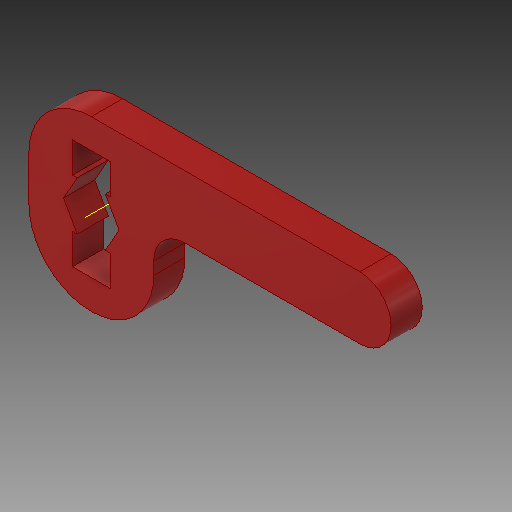
# Autodesk Inventor part: В. шарн. - держатель соединителя
Saved by Autodesk Inventor 2018 (Build 220112000, 112)
## iProperties
Created: 2020-02-23
Part Number: В. шарн. - держатель соединителя
Material: Типовые
Document SubType Name: Modeling
Designer: Leancher
Density: 1 g/cm^3
Appearance: По умолчанию
Author: Leancher
Autodesk Inventor part; units mm, degrees
ref_plane "YZ Plane" through (0, 0, 0) normal (1, 0, 0) x (0, 1, 0)
ref_plane "XZ Plane" through (0, 0, 0) normal (0, 1, 0) x (-1, 0, 0)
ref_plane "XY Plane" through (0, 0, 0) normal (0, 0, 1) x (1, 0, 0)
sketch "Эскиз1" plane through (0, 0, 0) normal (0, 0, 1) x (1, 0, 0)
  arc A0 (5.088, 16.8311) -> (-4.912, 6.8311) centre (5.088, 6.8311) ccw
  line L0 (7.3397, 7.2282) -> (8.088, 7.2282)
  line L1 (7.3397, 7.2282) -> (9.538, 3.3282)
  line L2 (2.8364, 7.2282) -> (0.638, 3.3282)
  line L3 (7.3397, -0.5718) -> (9.538, 3.3282)
  line L4 (2.8364, -0.5718) -> (0.638, 3.3282)
  line L5 (2.0673, 12.1282) -> (8.088, 12.1282)
  line L6 (8.088, 12.1282) -> (8.088, 7.2282)
  line L7 (2.088, 7.2282) -> (2.8364, 7.2282)
  line L8 (2.088, 12.1282) -> (2.088, 7.2282)
  line L9 (-4.912, 6.8311) -> (-4.912, -0.1747)
  arc A1 (-4.912, -0.1747) -> (15.088, -0.1747) centre (5.088, -0.1747) ccw
  line L10 (15.088, -0.1747) -> (15.088, 1.8311)
  line L11 (7.3397, -0.5718) -> (8.088, -0.5718)
  line L12 (2.088, -5.4718) -> (8.088, -5.4718)
  line L13 (8.088, -5.4718) -> (8.088, -0.5718)
  line L14 (2.088, -0.5718) -> (2.8364, -0.5718)
  line L15 (2.088, -5.4718) -> (2.088, -0.5718)
  line L16 (5.088, 16.8311) -> (48.088, 16.8311)
  line L17 (48.088, 6.8311) -> (20.088, 6.8311)
  arc A2 (53.088, 11.8311) -> (48.088, 16.8311) centre (48.088, 11.8311) ccw
  arc A3 (48.088, 6.8311) -> (53.088, 11.8311) centre (48.088, 11.8311) ccw
  arc A4 (20.088, 6.8311) -> (15.088, 1.8311) centre (20.088, 1.8311) ccw
  point P0 (5.088, 3.3282)
  constraints: 37 end point, 10 point on circle, 5 centre point, 1 point on line
extrude "Выдавливание1" add sketch "Эскиз1" along normal blind 5
